Autodesk Fusion 360 part; units mm, degrees
(part 2 of 2)
  spline S156 degree 3 poles (-2.409, -2.6721) (-2.1222, -2.8722) (-1.8693, -3.0094) (-1.6031, -3.1091) knots 0 0 0 0 1 1 1 1
  spline S157 degree 3 poles (-1.6031, -3.1091) (-1.4498, -3.1665) (-1.2489, -3.2213) (-0.935, -3.2912) knots 0 0 0 0 1 1 1 1
  spline S158 degree 3 poles (-0.935, -3.2912) (-0.6023, -3.3652) (-0.4933, -3.3954) (-0.4018, -3.4386) knots 0 0 0 0 1 1 1 1
  spline S159 degree 3 poles (-0.4018, -3.4386) (-0.285, -3.4938) (-0.2563, -3.5496) (-0.2988, -3.6392) knots 0 0 0 0 1 1 1 1
  spline S160 degree 3 poles (-0.2988, -3.6392) (-0.3058, -3.654) (-0.3376, -3.7016) (-0.3693, -3.745) knots 0 0 0 0 1 1 1 1
  spline S161 degree 3 poles (-0.3693, -3.745) (-0.4011, -3.7884) (-0.4577, -3.8789) (-0.4951, -3.946) knots 0 0 0 0 1 1 1 1
  spline S162 degree 3 poles (-0.4951, -3.946) (-0.5907, -4.1175) (-0.6284, -4.1744) (-0.6773, -4.2209) knots 0 0 0 0 1 1 1 1
  spline S163 degree 3 poles (-0.6773, -4.2209) (-0.7599, -4.2997) (-0.8244, -4.3055) (-0.9437, -4.2451) knots 0 0 0 0 1 1 1 1
  spline S164 degree 3 poles (-0.9437, -4.2451) (-0.9829, -4.2253) (-1.0546, -4.1863) (-1.1031, -4.1585) knots 0 0 0 0 1 1 1 1
  spline S165 degree 3 poles (-1.1031, -4.1585) (-1.1516, -4.1308) (-1.1929, -4.1097) (-1.195, -4.1117) knots 0 0 0 0 1 1 1 1
  spline S166 degree 3 poles (-1.195, -4.1117) (-1.2007, -4.1175) (-1.1403, -4.3146) (-1.0954, -4.437) knots 0 0 0 0 1 1 1 1
  spline S167 degree 3 poles (-1.0954, -4.437) (-1.0121, -4.6637) (-0.9214, -4.8374) (-0.8398, -4.9265) knots 0 0 0 0 1 1 1 1
  spline S168 degree 3 poles (-0.8398, -4.9265) (-0.7576, -5.0162) (-0.6987, -5.0344) (-0.6357, -4.9895) knots 0 0 0 0 1 1 1 1
  spline S169 degree 3 poles (0.9623, -3.4845) (0.9309, -3.4632) (0.9047, -3.4264) (0.874, -3.3605) knots 0 0 0 0 1 1 1 1
  spline S170 degree 3 poles (0.874, -3.3605) (0.8523, -3.314) (0.8517, -3.3099) (0.8617, -3.286) knots 0 0 0 0 1 1 1 1
  spline S171 degree 3 poles (0.8617, -3.286) (0.8846, -3.2311) (0.9454, -3.2121) (0.9967, -3.2438) knots 0 0 0 0 1 1 1 1
  spline S172 degree 3 poles (0.9967, -3.2438) (1.0445, -3.2733) (1.077, -3.3761) (1.0593, -3.4418) knots 0 0 0 0 1 1 1 1
  spline S173 degree 3 poles (1.0593, -3.4418) (1.0431, -3.5018) (1.0096, -3.5166) (0.9623, -3.4845) knots 0 0 0 0 1 1 1 1
  spline S174 degree 3 poles (0.6993, -3.0134) (0.6825, -3.0094) (0.6566, -2.9955) (0.6417, -2.9824) knots 0 0 0 0 1 1 1 1
  spline S175 degree 3 poles (0.6417, -2.9824) (0.6191, -2.9626) (0.6132, -2.9511) (0.6064, -2.9137) knots 0 0 0 0 1 1 1 1
  spline S176 degree 3 poles (0.6064, -2.9137) (0.597, -2.8619) (0.6023, -2.8228) (0.6221, -2.7983) knots 0 0 0 0 1 1 1 1
  spline S177 degree 3 poles (0.6221, -2.7983) (0.6428, -2.7728) (0.6945, -2.7755) (0.7587, -2.8056) knots 0 0 0 0 1 1 1 1
  spline S178 degree 3 poles (0.7587, -2.8056) (0.8731, -2.8592) (0.916, -2.9234) (0.8703, -2.9727) knots 0 0 0 0 1 1 1 1
  spline S179 degree 3 poles (0.8703, -2.9727) (0.8359, -3.0099) (0.7604, -3.0278) (0.6993, -3.0134) knots 0 0 0 0 1 1 1 1
  spline S180 degree 3 poles (0.5946, -2.6541) (0.5761, -2.6467) (0.5547, -2.5897) (0.5467, -2.5266) knots 0 0 0 0 1 1 1 1
  spline S181 degree 3 poles (0.5467, -2.5266) (0.5387, -2.4629) (0.5387, -2.4622) (0.56, -2.4231) knots 0 0 0 0 1 1 1 1
  spline S182 degree 3 poles (0.56, -2.4231) (0.5931, -2.3623) (0.6871, -2.2967) (0.741, -2.2967) knots 0 0 0 0 1 1 1 1
  spline S183 degree 3 poles (0.741, -2.2967) (0.8002, -2.2967) (0.837, -2.3481) (0.837, -2.4307) knots 0 0 0 0 1 1 1 1
  spline S184 degree 3 poles (0.837, -2.4307) (0.837, -2.5018) (0.8139, -2.5433) (0.7458, -2.5946) knots 0 0 0 0 1 1 1 1
  spline S185 degree 3 poles (0.7458, -2.5946) (0.665, -2.6554) (0.6311, -2.6688) (0.5946, -2.6541) knots 0 0 0 0 1 1 1 1
  spline S186 degree 3 poles (1.1787, -2.0595) (1.0812, -2.0468) (1.0113, -2.0162) (1.0029, -1.9826) knots 0 0 0 0 1 1 1 1
  spline S187 degree 3 poles (1.0029, -1.9826) (0.9956, -1.9535) (1.0037, -1.9337) (1.0456, -1.8783) knots 0 0 0 0 1 1 1 1
  spline S188 degree 3 poles (1.0456, -1.8783) (1.149, -1.7416) (1.2245, -1.7051) (1.2652, -1.7719) knots 0 0 0 0 1 1 1 1
  spline S189 degree 3 poles (1.2652, -1.7719) (1.2728, -1.7845) (1.2832, -1.8154) (1.2882, -1.8405) knots 0 0 0 0 1 1 1 1
  spline S190 degree 3 poles (1.2882, -1.8405) (1.298, -1.89) (1.3011, -2.0451) (1.2926, -2.0589) knots 0 0 0 0 1 1 1 1
  spline S191 degree 3 poles (1.2926, -2.0589) (1.2867, -2.0684) (1.2487, -2.0686) (1.1787, -2.0595) knots 0 0 0 0 1 1 1 1
  spline S192 degree 3 poles (-1.2819, -2.0356) (-1.3388, -2.0085) (-1.3954, -1.9418) (-1.4456, -1.8427) knots 0 0 0 0 1 1 1 1
  line L9 (-1.4456, -1.8427) -> (-1.4886, -1.758)
  line L10 (-1.4886, -1.758) -> (-1.5472, -1.7494)
  spline S193 degree 3 poles (-1.5472, -1.7494) (-1.7294, -1.7228) (-1.8197, -1.6353) (-1.7857, -1.5183) knots 0 0 0 0 1 1 1 1
  spline S194 degree 3 poles (-1.7857, -1.5183) (-1.7723, -1.472) (-1.7441, -1.4421) (-1.6148, -1.3367) knots 0 0 0 0 1 1 1 1
  spline S195 degree 3 poles (-1.6148, -1.3367) (-1.57, -1.3002) (-1.4882, -1.2259) (-1.4329, -1.1715) knots 0 0 0 0 1 1 1 1
  spline S196 degree 3 poles (-1.4329, -1.1715) (-1.343, -1.0831) (-1.3292, -1.066) (-1.3018, -1.0098) knots 0 0 0 0 1 1 1 1
  spline S197 degree 3 poles (-1.3018, -1.0098) (-1.2163, -0.8341) (-1.1224, -0.4455) (-0.8936, 0.6803) knots 0 0 0 0 1 1 1 1
  spline S198 degree 3 poles (-0.8936, 0.6803) (-0.8647, 0.8226) (-0.8378, 0.9474) (-0.8338, 0.9576) knots 0 0 0 0 1 1 1 1
  spline S199 degree 3 poles (-0.8338, 0.9576) (-0.8299, 0.9678) (-0.805, 0.9944) (-0.7785, 1.0168) knots 0 0 0 0 1 1 1 1
  spline S200 degree 3 poles (-0.7785, 1.0168) (-0.661, 1.1162) (-0.593, 1.1163) (-0.5793, 1.0169) knots 0 0 0 0 1 1 1 1
  spline S201 degree 3 poles (-0.5793, 1.0169) (-0.5654, 0.9154) (-0.6287, 0.6568) (-0.8385, -0.0417) knots 0 0 0 0 1 1 1 1
  spline S202 degree 3 poles (-0.8385, -0.0417) (-0.9587, -0.4418) (-1.2037, -1.2178) (-1.2188, -1.2459) knots 0 0 0 0 1 1 1 1
  spline S203 degree 3 poles (-1.2188, -1.2459) (-1.2225, -1.2529) (-1.2399, -1.2628) (-1.2575, -1.268) knots 0 0 0 0 1 1 1 1
  spline S204 degree 3 poles (-1.2575, -1.268) (-1.3741, -1.3025) (-1.5834, -1.4044) (-1.6308, -1.4499) knots 0 0 0 0 1 1 1 1
  spline S205 degree 3 poles (-1.6308, -1.4499) (-1.67, -1.4874) (-1.6726, -1.5106) (-1.6407, -1.5374) knots 0 0 0 0 1 1 1 1
  spline S206 degree 3 poles (-1.6407, -1.5374) (-1.6068, -1.566) (-1.5521, -1.5742) (-1.4626, -1.5644) knots 0 0 0 0 1 1 1 1
  spline S207 degree 3 poles (-1.4626, -1.5644) (-1.3262, -1.5494) (-1.3018, -1.5634) (-1.2928, -1.6622) knots 0 0 0 0 1 1 1 1
  spline S208 degree 3 poles (-1.2928, -1.6622) (-1.2827, -1.7729) (-1.2599, -1.8233) (-1.2199, -1.8233) knots 0 0 0 0 1 1 1 1
  spline S209 degree 3 poles (-1.2199, -1.8233) (-1.1742, -1.8233) (-1.1339, -1.7522) (-1.0893, -1.5923) knots 0 0 0 0 1 1 1 1
  spline S210 degree 3 poles (-1.0893, -1.5923) (-1.0686, -1.5184) (-1.0421, -1.4657) (-1.0196, -1.4536) knots 0 0 0 0 1 1 1 1
  spline S211 degree 3 poles (-1.0196, -1.4536) (-0.9579, -1.4206) (-0.8712, -1.487) (-0.774, -1.642) knots 0 0 0 0 1 1 1 1
  spline S212 degree 3 poles (-0.774, -1.642) (-0.7523, -1.6765) (-0.7299, -1.7048) (-0.7242, -1.7048) knots 0 0 0 0 1 1 1 1
  spline S213 degree 3 poles (-0.7242, -1.7048) (-0.7052, -1.7051) (-0.6661, -1.6688) (-0.6503, -1.6363) knots 0 0 0 0 1 1 1 1
  spline S214 degree 3 poles (-0.6503, -1.6363) (-0.6093, -1.5516) (-0.6449, -1.4573) (-0.7681, -1.3237) knots 0 0 0 0 1 1 1 1
  spline S215 degree 3 poles (-0.7681, -1.3237) (-0.8515, -1.2334) (-0.8795, -1.1909) (-0.9011, -1.1217) knots 0 0 0 0 1 1 1 1
  spline S216 degree 3 poles (-0.9011, -1.1217) (-0.9553, -0.9487) (-0.9057, -0.7143) (-0.7367, -0.3447) knots 0 0 0 0 1 1 1 1
  spline S217 degree 3 poles (-0.7367, -0.3447) (-0.704, -0.2732) (-0.6612, -0.1794) (-0.6416, -0.1362) knots 0 0 0 0 1 1 1 1
  spline S218 degree 3 poles (-0.6416, -0.1362) (-0.6221, -0.0931) (-0.5991, -0.0304) (-0.5905, 0.003) knots 0 0 0 0 1 1 1 1
  spline S219 degree 3 poles (-0.5905, 0.003) (-0.5727, 0.0729) (-0.5329, 0.2025) (-0.4316, 0.5212) knots 0 0 0 0 1 1 1 1
  spline S220 degree 3 poles (-0.4316, 0.5212) (-0.3921, 0.6453) (-0.3523, 0.775) (-0.3432, 0.8094) knots 0 0 0 0 1 1 1 1
  spline S221 degree 3 poles (-0.3432, 0.8094) (-0.323, 0.8854) (-0.3081, 0.8997) (-0.2439, 0.9043) knots 0 0 0 0 1 1 1 1
  spline S222 degree 3 poles (-0.2439, 0.9043) (-0.1692, 0.9097) (-0.1116, 0.8722) (-0.0885, 0.803) knots 0 0 0 0 1 1 1 1
  spline S223 degree 3 poles (-0.0885, 0.803) (-0.0756, 0.7645) (-0.0785, 0.6651) (-0.0945, 0.5985) knots 0 0 0 0 1 1 1 1
  spline S224 degree 3 poles (-0.0945, 0.5985) (-0.1288, 0.4554) (-0.235, 0.1821) (-0.4854, -0.407) knots 0 0 0 0 1 1 1 1
  spline S225 degree 3 poles (-0.4854, -0.407) (-0.7048, -0.9231) (-0.7515, -1.0449) (-0.743, -1.0789) knots 0 0 0 0 1 1 1 1
  spline S226 degree 3 poles (-0.743, -1.0789) (-0.7382, -1.0977) (-0.7081, -1.139) (-0.583, -1.2982) knots 0 0 0 0 1 1 1 1
  spline S227 degree 3 poles (-0.583, -1.2982) (-0.4949, -1.4103) (-0.4562, -1.4843) (-0.4518, -1.5492) knots 0 0 0 0 1 1 1 1
  line L11 (-0.4518, -1.5492) -> (-0.4484, -1.5977)
  line L12 (-0.4484, -1.5977) -> (-0.509, -1.6976)
  spline S228 degree 3 poles (-0.509, -1.6976) (-0.5423, -1.7525) (-0.5823, -1.8144) (-0.5979, -1.8351) knots 0 0 0 0 1 1 1 1
  spline S229 degree 3 poles (-0.5979, -1.8351) (-0.6255, -1.8719) (-0.6639, -1.8974) (-0.6914, -1.8971) knots 0 0 0 0 1 1 1 1
  spline S230 degree 3 poles (-0.6914, -1.8971) (-0.7224, -1.8967) (-0.7734, -1.8641) (-0.8315, -1.8074) knots 0 0 0 0 1 1 1 1
  line L13 (-0.8315, -1.8074) -> (-0.8931, -1.7472)
  line L14 (-0.8931, -1.7472) -> (-0.9063, -1.7717)
  spline S231 degree 3 poles (-0.9063, -1.7717) (-0.9431, -1.8396) (-1.0092, -1.9295) (-1.0515, -1.9691) knots 0 0 0 0 1 1 1 1
  spline S232 degree 3 poles (-1.0515, -1.9691) (-1.136, -2.0481) (-1.2107, -2.0696) (-1.2819, -2.0356) knots 0 0 0 0 1 1 1 1
  spline S233 degree 3 poles (1.0191, -1.0208) (0.9576, -0.9995) (0.9006, -0.9201) (0.86, -0.799) knots 0 0 0 0 1 1 1 1
  spline S234 degree 3 poles (0.86, -0.799) (0.8308, -0.712) (0.8323, -0.7102) (0.9353, -0.7102) knots 0 0 0 0 1 1 1 1
  spline S235 degree 3 poles (0.9353, -0.7102) (1.0085, -0.7102) (1.0125, -0.7111) (1.0626, -0.738) knots 0 0 0 0 1 1 1 1
  spline S236 degree 3 poles (1.0626, -0.738) (1.2339, -0.8298) (1.2549, -0.9404) (1.1144, -1.0113) knots 0 0 0 0 1 1 1 1
  spline S237 degree 3 poles (1.1144, -1.0113) (1.0799, -1.0286) (1.0504, -1.0316) (1.0191, -1.0208) knots 0 0 0 0 1 1 1 1
  spline S238 degree 3 poles (0.0789, 2.316) (-0.0724, 2.3342) (-0.2224, 2.3702) (-0.4165, 2.4348) knots 0 0 0 0 1 1 1 1
  spline S239 degree 3 poles (-0.4165, 2.4348) (-0.5884, 2.4919) (-0.6085, 2.5057) (-0.6641, 2.6046) knots 0 0 0 0 1 1 1 1
  spline S240 degree 3 poles (-0.6641, 2.6046) (-0.682, 2.6364) (-0.7112, 2.6845) (-0.7291, 2.7116) knots 0 0 0 0 1 1 1 1
  spline S241 degree 3 poles (-0.7291, 2.7116) (-0.7653, 2.7666) (-0.7647, 2.7525) (-0.7372, 2.8943) knots 0 0 0 0 1 1 1 1
  spline S242 degree 3 poles (-0.7372, 2.8943) (-0.6851, 3.1626) (-0.5618, 3.4008) (-0.413, 3.5206) knots 0 0 0 0 1 1 1 1
  spline S243 degree 3 poles (-0.413, 3.5206) (-0.2496, 3.6523) (-0.0732, 3.682) (0.1936, 3.6229) knots 0 0 0 0 1 1 1 1
  spline S244 degree 3 poles (0.1936, 3.6229) (0.4855, 3.5582) (0.697, 3.4394) (0.8004, 3.282) knots 0 0 0 0 1 1 1 1
  spline S245 degree 3 poles (0.8004, 3.282) (0.8491, 3.208) (0.8673, 3.1519) (0.872, 3.0614) knots 0 0 0 0 1 1 1 1
  spline S246 degree 3 poles (0.872, 3.0614) (0.8785, 2.9363) (0.843, 2.8293) (0.7478, 2.6873) knots 0 0 0 0 1 1 1 1
  spline S247 degree 3 poles (0.7478, 2.6873) (0.5778, 2.4336) (0.4796, 2.3536) (0.2995, 2.3222) knots 0 0 0 0 1 1 1 1
  spline S248 degree 3 poles (0.2995, 2.3222) (0.2419, 2.3121) (0.1357, 2.3091) (0.0789, 2.316) knots 0 0 0 0 1 1 1 1
  spline S249 degree 3 poles (0.3695, 2.5332) (0.4795, 2.5511) (0.5458, 2.5953) (0.5865, 2.678) knots 0 0 0 0 1 1 1 1
  spline S250 degree 3 poles (0.5865, 2.678) (0.6073, 2.7203) (0.6106, 2.7354) (0.6136, 2.8022) knots 0 0 0 0 1 1 1 1
  spline S251 degree 3 poles (0.6136, 2.8022) (0.6174, 2.8884) (0.6056, 2.9613) (0.5701, 3.0692) knots 0 0 0 0 1 1 1 1
  spline S252 degree 3 poles (0.5701, 3.0692) (0.5223, 3.2147) (0.4089, 3.407) (0.3608, 3.4239) knots 0 0 0 0 1 1 1 1
  spline S253 degree 3 poles (0.3608, 3.4239) (0.3212, 3.4379) (0.3197, 3.4078) (0.3533, 3.2689) knots 0 0 0 0 1 1 1 1
  spline S254 degree 3 poles (0.3533, 3.2689) (0.4005, 3.0738) (0.377, 2.94) (0.2773, 2.8354) knots 0 0 0 0 1 1 1 1
  spline S255 degree 3 poles (0.2773, 2.8354) (0.1834, 2.737) (0.0356, 2.6811) (-0.1635, 2.6688) knots 0 0 0 0 1 1 1 1
  spline S256 degree 3 poles (-0.1635, 2.6688) (-0.2162, 2.6655) (-0.2424, 2.6611) (-0.2406, 2.6557) knots 0 0 0 0 1 1 1 1
  spline S257 degree 3 poles (-0.2406, 2.6557) (-0.2349, 2.6381) (0.0027, 2.5651) (0.1196, 2.5451) knots 0 0 0 0 1 1 1 1
  spline S258 degree 3 poles (0.1196, 2.5451) (0.2423, 2.5241) (0.2974, 2.5215) (0.3695, 2.5332) knots 0 0 0 0 1 1 1 1
  spline S259 degree 3 poles (-3.3528, -4.2207) (-3.2798, -4.1858) (-3.1635, -4.0944) (-2.9988, -3.9424) knots 0 0 0 0 1 1 1 1
  spline S260 degree 3 poles (-2.9988, -3.9424) (-2.8198, -3.777) (-2.4546, -3.4053) (-2.2585, -3.1886) knots 0 0 0 0 1 1 1 1
  spline S261 degree 3 poles (-2.2585, -3.1886) (-2.202, -3.1263) (-2.2002, -3.123) (-2.2141, -3.1128) knots 0 0 0 0 1 1 1 1
  spline S262 degree 3 poles (-2.2141, -3.1128) (-2.2221, -3.107) (-2.2831, -3.0687) (-2.3496, -3.0277) knots 0 0 0 0 1 1 1 1
  spline S263 degree 3 poles (-2.3496, -3.0277) (-2.4505, -2.9657) (-2.4722, -2.955) (-2.4801, -2.9634) knots 0 0 0 0 1 1 1 1
  spline S264 degree 3 poles (-2.4801, -2.9634) (-2.4854, -2.9689) (-2.5438, -3.0433) (-2.6101, -3.1287) knots 0 0 0 0 1 1 1 1
  spline S265 degree 3 poles (-2.6101, -3.1287) (-2.9159, -3.5232) (-3.122, -3.7537) (-3.1689, -3.7537) knots 0 0 0 0 1 1 1 1
  spline S266 degree 3 poles (-3.1689, -3.7537) (-3.19, -3.7537) (-3.2627, -3.6827) (-3.4505, -3.4786) knots 0 0 0 0 1 1 1 1
  spline S267 degree 3 poles (-3.4505, -3.4786) (-3.5609, -3.3586) (-3.6722, -3.2413) (-3.698, -3.2179) knots 0 0 0 0 1 1 1 1
  spline S268 degree 3 poles (-3.698, -3.2179) (-3.7928, -3.1317) (-3.8392, -3.1116) (-3.8494, -3.1523) knots 0 0 0 0 1 1 1 1
  spline S269 degree 3 poles (-3.8494, -3.1523) (-3.8625, -3.2047) (-3.7948, -3.511) (-3.7215, -3.7307) knots 0 0 0 0 1 1 1 1
  spline S270 degree 3 poles (-3.7215, -3.7307) (-3.6147, -4.0509) (-3.4998, -4.2407) (-3.412, -4.2417) knots 0 0 0 0 1 1 1 1
  spline S271 degree 3 poles (-3.412, -4.2417) (-3.4039, -4.2417) (-3.3772, -4.2323) (-3.3528, -4.2207) knots 0 0 0 0 1 1 1 1
  spline S272 degree 3 poles (3.3031, -2.7354) (3.4328, -2.7033) (3.4923, -2.6301) (3.483, -2.5143) knots 0 0 0 0 1 1 1 1
  spline S273 degree 3 poles (3.483, -2.5143) (3.478, -2.4524) (3.432, -2.3552) (3.3661, -2.2671) knots 0 0 0 0 1 1 1 1
  spline S274 degree 3 poles (3.3661, -2.2671) (3.3402, -2.2325) (3.2532, -2.1374) (3.1727, -2.0558) knots 0 0 0 0 1 1 1 1
  spline S275 degree 3 poles (3.1727, -2.0558) (3.0922, -1.9741) (3.0263, -1.9034) (3.0263, -1.8986) knots 0 0 0 0 1 1 1 1
  spline S276 degree 3 poles (3.0263, -1.8986) (3.0263, -1.8859) (3.0395, -1.8877) (3.1008, -1.9088) knots 0 0 0 0 1 1 1 1
  spline S277 degree 3 poles (3.1008, -1.9088) (3.4601, -2.0322) (3.706, -1.9604) (3.6352, -1.7526) knots 0 0 0 0 1 1 1 1
  spline S278 degree 3 poles (3.6352, -1.7526) (3.6111, -1.682) (3.5123, -1.6088) (3.441, -1.6088) knots 0 0 0 0 1 1 1 1
  spline S279 degree 3 poles (3.441, -1.6088) (3.3611, -1.6088) (3.2134, -1.5626) (3.0855, -1.4974) knots 0 0 0 0 1 1 1 1
  spline S280 degree 3 poles (3.0855, -1.4974) (2.9881, -1.4479) (2.839, -1.3531) (2.8427, -1.343) knots 0 0 0 0 1 1 1 1
  spline S281 degree 3 poles (2.8427, -1.343) (2.844, -1.3392) (3.0165, -1.1574) (3.226, -0.9389) knots 0 0 0 0 1 1 1 1
  spline S282 degree 3 poles (3.226, -0.9389) (3.7535, -0.3887) (3.7766, -0.3629) (3.8806, -0.2073) knots 0 0 0 0 1 1 1 1
  spline S283 degree 3 poles (3.8806, -0.2073) (4.0663, 0.0705) (4.0967, 0.3077) (3.9656, 0.4566) knots 0 0 0 0 1 1 1 1
  spline S284 degree 3 poles (3.9656, 0.4566) (3.8886, 0.5441) (3.7533, 0.5881) (3.6733, 0.5518) knots 0 0 0 0 1 1 1 1
  spline S285 degree 3 poles (3.6733, 0.5518) (3.6485, 0.5405) (3.6361, 0.5259) (3.5993, 0.4651) knots 0 0 0 0 1 1 1 1
  spline S286 degree 3 poles (3.5993, 0.4651) (3.544, 0.3736) (3.4297, 0.2214) (3.322, 0.096) knots 0 0 0 0 1 1 1 1
  spline S287 degree 3 poles (3.322, 0.096) (3.0564, -0.2135) (2.5426, -0.7126) (2.0814, -1.1092) knots 0 0 0 0 1 1 1 1
  spline S288 degree 3 poles (2.0814, -1.1092) (2.0438, -1.1415) (2.013, -1.1722) (2.013, -1.1775) knots 0 0 0 0 1 1 1 1
  spline S289 degree 3 poles (2.013, -1.1775) (2.013, -1.1827) (2.0305, -1.1958) (2.0518, -1.2066) knots 0 0 0 0 1 1 1 1
  spline S290 degree 3 poles (2.0518, -1.2066) (2.1537, -1.2579) (2.2803, -1.3525) (2.3788, -1.4509) knots 0 0 0 0 1 1 1 1
  spline S291 degree 3 poles (2.3788, -1.4509) (2.5749, -1.6468) (2.7001, -1.8648) (2.7504, -2.0982) knots 0 0 0 0 1 1 1 1
  spline S292 degree 3 poles (2.7504, -2.0982) (2.7608, -2.1465) (2.7637, -2.1928) (2.7635, -2.3115) knots 0 0 0 0 1 1 1 1
  spline S293 degree 3 poles (2.7635, -2.3115) (2.7634, -2.4503) (2.7617, -2.4702) (2.7433, -2.5477) knots 0 0 0 0 1 1 1 1
  spline S294 degree 3 poles (2.7433, -2.5477) (2.7246, -2.6264) (2.7241, -2.6332) (2.7354, -2.6457) knots 0 0 0 0 1 1 1 1
  spline S295 degree 3 poles (2.7354, -2.6457) (2.7741, -2.6884) (2.9663, -2.7418) (3.1113, -2.7502) knots 0 0 0 0 1 1 1 1
  spline S296 degree 3 poles (3.1113, -2.7502) (3.1712, -2.7536) (3.256, -2.7471) (3.3031, -2.7354) knots 0 0 0 0 1 1 1 1
  spline S297 degree 3 poles (-1.5924, 3.3506) (-1.5126, 3.3714) (-1.4609, 3.4158) (-1.4291, 3.4908) knots 0 0 0 0 1 1 1 1
  spline S298 degree 3 poles (-1.4291, 3.4908) (-1.4122, 3.5306) (-1.4066, 3.6581) (-1.4186, 3.7266) knots 0 0 0 0 1 1 1 1
  spline S299 degree 3 poles (-1.4186, 3.7266) (-1.4388, 3.8413) (-1.4985, 3.9902) (-1.5445, 4.0406) knots 0 0 0 0 1 1 1 1
  spline S300 degree 3 poles (-1.5445, 4.0406) (-1.5812, 4.0808) (-1.5851, 4.0721) (-1.5856, 3.9487) knots 0 0 0 0 1 1 1 1
  spline S301 degree 3 poles (-1.5856, 3.9487) (-1.5859, 3.8652) (-1.5892, 3.8276) (-1.5992, 3.794) knots 0 0 0 0 1 1 1 1
  spline S302 degree 3 poles (-1.5992, 3.794) (-1.643, 3.647) (-1.758, 3.5253) (-1.9323, 3.4417) knots 0 0 0 0 1 1 1 1
  spline S303 degree 3 poles (-1.9323, 3.4417) (-1.9672, 3.4249) (-1.9957, 3.4085) (-1.9957, 3.4051) knots 0 0 0 0 1 1 1 1
  spline S304 degree 3 poles (-1.9957, 3.4051) (-1.9957, 3.3948) (-1.8614, 3.3579) (-1.7738, 3.3441) knots 0 0 0 0 1 1 1 1
  spline S305 degree 3 poles (-1.7738, 3.3441) (-1.7272, 3.3367) (-1.6325, 3.3401) (-1.5924, 3.3506) knots 0 0 0 0 1 1 1 1
sketch "Sketch24" plane through (0, 0, 5.46) normal (0, 0, 1) x (-1, 0, 0)
  arc A0 (7.029, 4.3192) -> (6.15, 5.4991) centre (0, 0) ccw
  arc A1 (6.15, 5.4991) -> (-6.15, 5.4991) centre (0, 0) ccw
  arc A2 (-6.15, 5.4991) -> (-7.029, 4.3192) centre (0, 0) ccw
  line L0 (6.15, 5.4991) -> (0, 0)
  line L1 (0, 0) -> (-6.15, 5.4991)
  constraint coincident A0.end A1.start
  constraint coincident A0.centre A1.centre
  constraint coincident A1.end A2.start
extrude "Extrude27" cut sketch "Sketch24" along normal up to surface (2 mm away) bodies 6
sketch "Sketch25" plane through (0, 0, 1.6) normal (0, 0, -1) x (1, 0, 0)
  circle A0 centre (0, 0) radius 8.25
  circle A1 centre (0, 0) radius 7.25
  circle A2 centre (0, 0) radius 7.25
  line L0 (0, 0) -> (12.5, 0) construction
  line L1 (0, 0) -> (0, -3.5) construction
  line L2 (0, 0) -> (0, 3) construction
  line L3 (12.5, -0.95) -> (0, -0.95)
  line L4 (12.5, 0.95) -> (0, 0.95)
  line L5 (6.35, -0.95) -> (6.35, 0.95)
  point P0 (8.25, 0)
  dimension "d182" = 0.95
  dimension "d183" = 0.95
  dimension "d184" = 1.9
  constraint coincident A0.centre A1.centre
  constraint horizontal L0
  constraint perpendicular L0 L1
  constraint perpendicular L0 L2
  constraint coincident L1 L3.end
  constraint perpendicular L1 L3
  constraint coincident L2 L4.end
  constraint perpendicular L2 L4
  constraint coincident L3 L5.start
  constraint perpendicular L3 L5
  constraint coincident L4 L5.end
  constraint coincident A0 P0
  constraint coincident L0 P0
  measures "d182" distance of L0 L3
  measures "d183" distance of L0 L4
  measures "d184" distance of L5 P0
extrude "Extrude28" cut sketch "Sketch25" against normal up to surface (2.56 mm away) contours A0 A1 A2 L3 L4 | A1 A2 L3 L4 L5 picked at (7.5349, 0.8448) picked at (6.65, 0) bodies 6
sketch "Sketch26" plane through (0, 0, 2.1) normal (0, 0, 1) x (-1, 0, 0)
  line L0 (-6.35, -0.95) -> (-7.1875, -0.95)
  line L1 (-6.35, 0.95) -> (-6.35, -0.95)
  line L2 (-7.1875, 0.95) -> (-6.35, 0.95)
  line L3 (-6.35, -0.95) -> (-5.85, -0.95)
  line L4 (-5.85, -0.95) -> (-5.85, 0.95)
  line L5 (-5.85, 0.95) -> (-6.35, 0.95)
  dimension "d188" = 0.5
  constraint coincident L0.start L1.end
  constraint perpendicular L1 L3
  constraint perpendicular L2 L4
  constraint coincident L1.start L2.end
  constraint perpendicular L1 L5
  measures "d188" distance of L0.start L3.end
extrude "Extrude29" add sketch "Sketch26" along normal up to surface (2.56 mm away) bodies 6
sketch "Sketch27" plane through (6.35, 0, 0) normal (1, 0, 0) x (0, 1, 0)
  line L0 (-0.95, 2.1) -> (-0.95, 1.6)
  line L1 (-0.95, 1.6) -> (0.95, 1.6)
  line L2 (0.95, 1.6) -> (0.95, 2.1)
  line L3 (0.95, 2.1) -> (0.95, 4.66)
  line L4 (0.95, 4.66) -> (-0.95, 4.66)
  line L5 (-0.95, 4.66) -> (-0.95, 2.1)
  line L6 (-0.95, 4.16) -> (0.95, 4.16)
  dimension "d191" = 0.5
  constraint coincident L5 L6.start
  constraint perpendicular L5 L6
  constraint coincident L3 L6.end
  measures "d191" distance of L4 L6
extrude "Extrude30" add sketch "Sketch27" along normal up to surface contours L3 L4 L5 L6 end surface at (7.5053, -1.932, 6.1267) on bodies 6 bodies 6
fillet "Fillet13" radius 0.5 3 edges at (6.35, 0, 1.6) (8.25, 0, 4.16) (6.35, 0, 4.16) on bodies 6
fillet "Fillet14" radius 1 1 edges at (5.85, 0, 4.66) on bodies 6
equation "d1 = 10.7 mm - 9.1 mm"
equation "d4 = ( 11 / 2 ) * 1 mm"
equation "d5 = d4"
equation "d11 = ( 11 / 2 ) * 1 mm"
equation "d12 = ( 11 / 2 ) * 1 mm"
equation "d14 = 2 mm - 1.25 mm"
equation "d23 = ( 15.2 / 2 ) * 1 mm"
equation "d43 = 16 mm + ( 0.5 / 2 ) * 1 mm"
equation "d47 = 10.7 mm - 3.74 mm + 20.8 mm - 10.7 mm"
equation "d75 = 2 mm - 1.24 mm - 0.5 mm"
equation "d78 = 9.1 mm - 3.24 mm"
equation "d156 = -1.24 mm + 0.5 mm"
equation "d182 = ( 1.9 / 2 ) * 1 mm"
equation "d183 = ( 1.9 / 2 ) * 1 mm"
